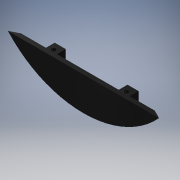
# Autodesk Inventor part: vs
Saved by Autodesk Inventor 2017 (Build 210142000, 142)
## iProperties
Part Number: vs
Material: Genérico
Document SubType Name: Modeling
Designer: Roberto
Density: 1 g/cm^3
Appearance: Valor por defecto
Author: Roberto
Autodesk Inventor part; units mm, degrees
ref_plane "YZ Plane" through (0, 0, 0) normal (1, 0, 0) x (0, 1, 0)
ref_plane "XZ Plane" through (0, 0, 0) normal (0, 1, 0) x (-1, 0, 0)
ref_plane "Plano de trabajo1" through (-3.6934, 0.2114, -2.9776) normal (-0.0004218, 0, -0.9999999) x (-0.9999997, -0.0005838, 0.0004218)
sketch "Boceto1" plane through (-3.6934, 0.2114, -2.9776) normal (-0.0004218, 0, -0.9999999) x (-0.9999997, -0.0005838, 0.0004218)
  line L0 (-3.0164, 1.9579) -> (1.1656, 1.9607) projected
  line L1 (0, 2.3193) -> (-2.3, 2.3193) projected
  line L2 (0, 2.3193) -> (-5.2081, 2.3193)
  line L3 (-5.2081, 2.3193) -> (-5.2081, 2.5193)
  line L4 (-5.2081, 2.5193) -> (5.9957, 2.5193)
  line L5 (5.9957, 2.5193) -> (5.9957, 2.3193)
  line L6 (0, 2.3193) -> (5.9957, 2.3193)
  point P0 (-3.692, -0.2136)
  dimension "d1" = 0.2
  dimension "d2" = 0.2
  constraints: 10 end point, 2 perpendicular, 2 point on line, 1 horizontal
  measures "d1" distance of L2.end L3.end
  measures "d2" distance of L4.end L5.end
extrude "Extrusión1" add sketch "Boceto1" along normal blind 3
ref_plane "Plano de trabajo2" through (-3.6921, 0.2114, 0.1224) normal (-0.0004218, 0, -0.9999999) x (-0.9999997, -0.0005838, 0.0004218)
sketch "Boceto2" plane through (-3.6921, 0.2114, 0.1224) normal (-0.0004218, 0, -0.9999999) x (-0.9999997, -0.0005838, 0.0004218)
  line L0 (-7.8545, -5.065) -> (-7.6172, -5.0078)
  line L1 (-6.9665, -8.3558) -> (-7.6172, -5.0078)
  line L2 (-7.6172, -5.0078) -> (-6.9665, -8.3558)
  line L3 (-7.2432, -8.3558) -> (-6.9376, -8.3558)
  line L4 (-7.2432, -8.3558) -> (-6.9376, -8.3558)
  line L5 (-6.9665, -8.3558) -> (-7.2432, -8.3558)
  line L6 (-7.8545, -5.065) -> (-7.2432, -8.3558)
  line L7 (-7.8545, -5.065) -> (-7.2432, -8.3558)
  line L8 (-7.2432, -8.3558) -> (7.7568, -8.3558)
  arc A0 (-3.3928, 3.2058) -> (-7.8545, -5.065) centre (0.4426, -4.202) ccw
  arc A1 (0.2568, 4.0292) -> (-3.3486, 2.956) centre (1.1532, -5.5745) ccw
  line L9 (0.2568, 4.2722) -> (0.2568, 4.0292)
  arc A2 (0.2568, 4.2722) -> (-3.3928, 3.2058) centre (1.1532, -5.5745) ccw
  arc A3 (-3.2814, 2.9912) -> (-7.6172, -5.0078) centre (0.4426, -4.202) ccw
  line L10 (0.2568, -8.3558) -> (0.2568, 10.2551)
  line L11 (0.2568, 4.2722) -> (-10.676, 4.2722)
  line L12 (-10.676, 4.2722) -> (-10.676, -8.3558)
  line L13 (-7.2432, -8.3558) -> (-10.676, -8.3558)
  line L14 (0.2568, 4.2722) -> (-10.676, 4.2722)
  line L15 (-10.676, 4.2722) -> (-10.676, -8.3558)
  line L16 (-10.676, -8.3558) -> (-7.2432, -8.3558)
  line L17 (-7.2432, -8.3558) -> (-7.8545, -5.065)
  point P0 (-3.692, -0.2136)
  dimension "d6" = 15
  constraints: 36 end point, 11 point on circle, 6 horizontal, 5 collinear, 4 centre point, 2 coincident, 2 vertical, 1 midpoint, 1 perpendicular
  measures "d6" distance of L8.start L8.end
revolve "Revolución1" cut sketch "Boceto2" angle 360 about axis through (-3.944, -8.1445, 0.1225) along (-0.0005838, 0.9999998, 0.0000002) contours A0 A2 L9 A1 A3 L0 | L6 L13 L12 L11 A2 A0
sketch "Boceto3" plane through (-6.9813, 2.7288, -2.9762) normal (-0.0005838, 0.9999998, 0.0000002) x (0.9999997, 0.0005838, -0.0004218)
  arc A0 (6.0592, 0) -> (0, 0) centre (3.0296, -3.1) ccw projected
  line L0 (6.0592, 0) -> (0, 0) projected
  line L1 (6.0592, 0) -> (0, 0) projected
  line L2 (3.0296, 0) -> (1.6296, 0)
  line L3 (1.6296, 0) -> (1.6296, 0.5)
  line L4 (1.6296, 0.5) -> (1.1296, 0.5)
  line L5 (1.1296, 0.5) -> (1.1296, 0)
  line L6 (1.1296, 0) -> (1.6296, 0)
  line L7 (3.0296, 0) -> (4.4296, 0)
  line L8 (4.4296, 0) -> (4.9296, 0)
  line L9 (4.9296, 0) -> (4.9296, 0.5)
  line L10 (4.9296, 0.5) -> (4.4296, 0.5)
  line L11 (4.4296, 0.5) -> (4.4296, 0)
  point P0 (6.9784, -2.9792)
  dimension "d8" = 1.4
  dimension "d9" = 0.5
  dimension "d10" = 0.5
  dimension "d11" = 0.5
  dimension "d12" = 1.4
  dimension "d13" = 0.5
  dimension "d14" = 0.5
  dimension "d15" = 0.5
  constraints: 20 end point, 6 point on line, 1 collinear, 1 midpoint, 1 perpendicular, 1 vertical
  measures "d8" distance of L2.start L2.end
  measures "d9" distance of L2.end L3.end
  measures "d10" distance of L3.end L4.end
  measures "d11" distance of L4.end L5.end
  measures "d12" distance of L2.start L7.end
  measures "d13" distance of L7.end L8.end
  measures "d14" distance of L8.end L9.end
  measures "d15" distance of L9.end L10.end
extrude "Extrusión2" add sketch "Boceto3" along normal blind 0.4 contours L0 L11 L10 L9 | L5 L4 L3 L0
sketch "Boceto4" plane through (-3.6934, 0.2114, -2.9776) normal (0.0004218, 0, 0.9999999) x (0.9999997, 0.0005838, -0.0004218)
  line L0 (2.7728, 2.5193) -> (1.6432, 2.5193) projected
  line L1 (1.6432, 2.5193) -> (1.6432, 2.9193) projected
  line L2 (1.1432, 2.9193) -> (1.6432, 2.9193) projected
  line L3 (1.1432, 2.5193) -> (1.1432, 2.9193) projected
  line L4 (1.1432, 2.5193) -> (-1.6568, 2.5193) projected
  line L5 (-1.6568, 2.5193) -> (-1.6568, 2.9193) projected
  line L6 (-2.1568, 2.9193) -> (-1.6568, 2.9193) projected
  line L7 (-2.1568, 2.5193) -> (-2.1568, 2.9193) projected
  line L8 (-2.1568, 2.5193) -> (-3.2864, 2.5193) projected
  line L9 (-3.6805, 2.3193) -> (3.1669, 2.3193) projected
  circle A0 centre (-1.9068, 2.6193) radius 0.1
  circle A1 centre (1.3932, 2.6193) radius 0.1
  point P0 (3.692, -0.2136)
  dimension "d18" = 0.2
  dimension "d19" = 0.2
  constraints: 2 centre point, 2 other
  measures "d18" diameter of A0
  measures "d19" diameter of A1
extrude "Extrusión3" cut sketch "Boceto4" against normal blind 0.3
